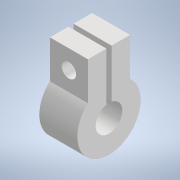
# Autodesk Inventor part: SetCollar_d6
Saved by Autodesk Inventor 2021 (Build 250183000, 183)
## iProperties
Created: 2020-10-10
Part Number: SetCollar_d6
Material: 一般
Document SubType Name: Modeling
Designer: yuta2
Density: 1 g/cm^3
Appearance: 青 - 壁塗料 - 光沢
Author: yuta2
Autodesk Inventor part; units mm, degrees
ref_plane "YZ Plane" through (0, 0, 0) normal (1, 0, 0) x (0, 1, 0)
ref_plane "XZ Plane" through (0, 0, 0) normal (0, 1, 0) x (-1, 0, 0)
ref_plane "XY Plane" through (0, 0, 0) normal (0, 0, 1) x (1, 0, 0)
sketch "スケッチ1" plane through (0, 0, 0) normal (1, 0, 0) x (0, 1, 0)
  circle A0 centre (0, 0) radius 3.15
  circle A1 centre (0, 0) radius 7.5
  line L0 (0, 0) -> (14.5902, 0)
  line L1 (14.5902, 5) -> (5.5902, 5)
  line L2 (5.5902, 5) -> (5.5902, -5)
  line L3 (5.5902, -5) -> (14.5902, -5)
  line L4 (14.5902, -5) -> (14.5902, 5)
  line L5 (14.5902, 0.6) -> (5.5902, 0.6)
  line L6 (5.5902, 0.6) -> (5.5902, -0.6)
  line L7 (5.5902, -0.6) -> (14.5902, -0.6)
  line L8 (14.5902, -0.6) -> (14.5902, 0.6)
  line L9 (5.5902, 0.6) -> (3.0923, 0.6)
  line L10 (5.5902, -0.6) -> (3.0923, -0.6)
  dimension "d1" = 15
  dimension "d0" = 6.3
  dimension "d2" = 1.2
  dimension "d3" = 9
  dimension "d4" = 10
  constraints: 22 end point, 5 parallel, 4 horizontal, 2 coincident, 2 perpendicular, 2 point on circle, 2 point on line, 1 centre point, 1 midpoint, 5 other
  measures "d0" diameter of A0
  measures "d2" distance between parallel lines of L7 L5
  measures "d3" distance of L2.end L3.end
  measures "d4" distance of L3.end L1.start
extrude "押し出し1" add sketch "スケッチ1" along normal blind 9 contours A0 L10 L2 A1 L9 | L2 A1 L5 | L7 A1 L2 | L1 L4 L5 A1 | A1 L7 L4 L3
sketch "スケッチ2" plane through (0, 5.5902, -5) normal (0, 0, -1) x (-1, 0, 0)
  line L0 (0, 9) -> (-9, 9) projected
  line L1 (-4.5, 9) -> (-4.5, 3.2578)
  point P0 (0, -5.5902)
  point P1 (-4.5, 4.5)
  dimension "d7" = 4.5
  constraints: 2 end point, 1 midpoint, 1 point on line, 1 vertical
  measures "d7" distance from line of L0 point (-4.5, 4.5)
hole "穴1" at (4.5, 10.0902, -5) direction (0, 0, 1) diameter 3.4 end through all
